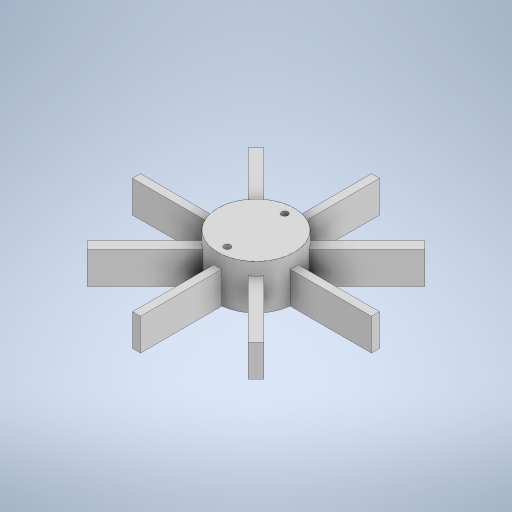
# Autodesk Inventor part: sweeper
Saved by Autodesk Inventor 2024 (Build 280153000, 153)
## iProperties
Created: 2024-05-20
Part Number: sweeper
Material: Generic
Document SubType Name: Modeling
Designer: ryana
Density: 1 g/cm^3
Appearance: Default
Author: ryana
Autodesk Inventor part; units mm, degrees
ref_plane "YZ Plane" through (0, 0, 0) normal (1, 0, 0) x (0, 1, 0)
ref_plane "XZ Plane" through (0, 0, 0) normal (0, 1, 0) x (-1, 0, 0)
ref_plane "XY Plane" through (0, 0, 0) normal (0, 0, 1) x (1, 0, 0)
sketch "Sketch2" plane through (0, 0, 0) normal (0, 1, 0) x (-1, 0, 0)
  circle A0 centre (0, 0) radius 12
  line L0 (-1.25, 37.5) -> (-1.25, -37.5)
  line L1 (-1.25, -37.5) -> (1.25, -37.5)
  line L2 (1.25, -37.5) -> (1.25, 37.5)
  line L3 (1.25, 37.5) -> (-1.25, 37.5)
  line L4 (-1.25, 37.5) -> (1.25, -37.5) construction
  line L5 (-1.25, -37.5) -> (1.25, 37.5) construction
  line L6 (-37.5, -1.25) -> (37.5, -1.25)
  line L7 (37.5, -1.25) -> (37.5, 1.25)
  line L8 (37.5, 1.25) -> (-37.5, 1.25)
  line L9 (-37.5, 1.25) -> (-37.5, -1.25)
  line L10 (-37.5, -1.25) -> (37.5, 1.25) construction
  line L11 (37.5, -1.25) -> (-37.5, 1.25) construction
  line L12 (1.25, 1.25) -> (-1.25, -1.25)
  line L13 (-1.25, -1.25) -> (25.2665, -27.7665)
  line L14 (25.2665, -27.7665) -> (27.7665, -25.2665)
  line L15 (27.7665, -25.2665) -> (1.25, 1.25)
  line L16 (1.25, 1.25) -> (-1.25, -1.25)
  line L17 (-1.25, -1.25) -> (-27.7665, 25.2665)
  line L18 (-27.7665, 25.2665) -> (-25.2665, 27.7665)
  line L19 (-25.2665, 27.7665) -> (1.25, 1.25)
  line L20 (-1.25, 1.25) -> (1.25, -1.25)
  line L21 (1.25, -1.25) -> (-25.2665, -27.7665)
  line L22 (-25.2665, -27.7665) -> (-27.7665, -25.2665)
  line L23 (-27.7665, -25.2665) -> (-1.25, 1.25)
  line L24 (-1.25, 1.25) -> (1.25, -1.25)
  line L25 (1.25, -1.25) -> (27.7665, 25.2665)
  line L26 (27.7665, 25.2665) -> (25.2665, 27.7665)
  line L27 (25.2665, 27.7665) -> (-1.25, 1.25)
  point P0 (7.1427, -9.6427)
  point P1 (9.6427, -7.1427)
  point P2 (11.9347, -1.25)
  point P3 (11.9347, 1.25)
  point P4 (9.6427, 7.1427)
  point P5 (7.1427, 9.6427)
  point P6 (1.25, 11.9347)
  point P7 (-1.25, 11.9347)
  point P8 (-7.1427, 9.6427)
  point P9 (-9.6427, 7.1427)
  point P10 (-11.9347, 1.25)
  point P11 (-11.9347, -1.25)
  point P12 (-9.6427, -7.1427)
  point P13 (-7.1427, -9.6427)
  point P14 (-1.25, -11.9347)
  point P15 (1.25, -11.9347)
  dimension "d0" = 24
  dimension "d1" = 75
  dimension "d2" = 2.5
  dimension "d3" = 75
  dimension "d4" = 2.5
  dimension "d5" = 37.5
  dimension "d6" = 37.5
  dimension "d7" = 37.5
  dimension "d8" = 37.5
  constraints: 56 end point, 12 parallel, 8 point on line, 6 perpendicular, 4 midpoint, 1 centre point, 1 coincident, 1 horizontal, 1 vertical
  measures "d0" diameter of A0
  measures "d1" distance of L0.start L0.end
  measures "d2" distance of L1.end L0.end
  measures "d3" distance of L6.start L6.end
  measures "d4" distance of L7.end L6.end
  measures "d5" distance of L13.end L12.end
  measures "d6" distance of L12.end L17.end
  measures "d7" distance of L20.end L21.end
  measures "d8" distance of L25.end L20.end
extrude "Extrusion1" add sketch "Sketch2" along normal blind 10
sketch "Sketch3" plane through (0, 10, 0) normal (0, 1, 0) x (1, 0, 0)
  circle A0 centre (0, 0) radius 12
  dimension "d11" = 24
  constraints: 1 centre point, 1 coincident
  measures "d11" diameter of A0
extrude "Extrusion2" add sketch "Sketch3" along normal blind 4
sketch "Sketch4" plane through (0, 14, 0) normal (0, 1, 0) x (1, 0, 0)
  line L0 (0, 0) -> (0, 12)
  line L1 (1.25, 11.9347) -> (1.25, 37.5) projected
  line L2 (0, 0) -> (12, 0) construction
  line L3 (0, 12) -> (0, -12)
  line L4 (0, -12) -> (0, -9)
  line L5 (0, -12) -> (3, -12) construction
  line L6 (0, 12) -> (0, 9)
  line L7 (0, 12) -> (3, 12) construction
  circle A0 centre (0, -9) radius 1
  circle A1 centre (0, 9) radius 1
  dimension "d14" = 12
  dimension "d15" = 90
  dimension "d16" = 24
  dimension "d17" = 0
  dimension "d18" = 3
  dimension "d19" = 90
  dimension "d20" = 3
  dimension "d21" = 90
  dimension "d22" = 2
  dimension "d23" = 2
  constraints: 14 end point, 3 collinear, 3 horizontal, 3 perpendicular, 2 centre point, 2 coincident, 1 parallel
  measures "d14" distance of L0.start L0.end
  measures "d15" angle of L2 L0
  measures "d16" distance of L0.end L3.end
  measures "d17" distance between parallel lines of L3 L0
  measures "d18" distance of L3.end L4.end
  measures "d19" angle of L5 L4
  measures "d20" distance of L0.end L6.end
  measures "d21" angle of L6 L7
  measures "d22" diameter of A0
  measures "d23" diameter of A1
extrude "Extrusion3" cut sketch "Sketch4" against normal blind 20
body "Solid1"
